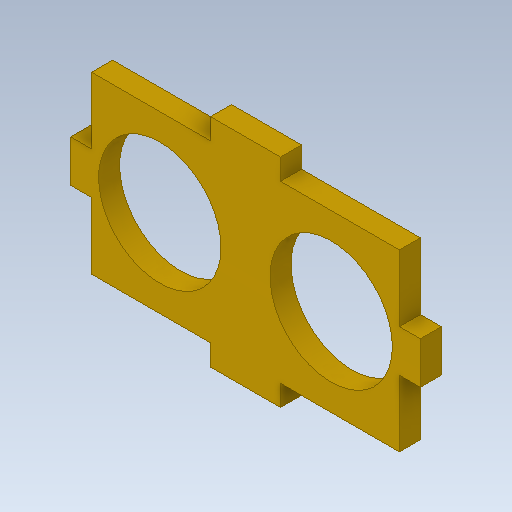
# Autodesk Inventor part: Part5
Saved by Autodesk Inventor 2020 (Build 240168000, 168)
## iProperties
Created: 2020-03-11
Part Number: Part5
Material: Generic
Document SubType Name: Modeling
Designer: tor16003
Density: 1 g/cm^3
Appearance: Gold
Author: tor16003
Autodesk Inventor part; units mm, degrees
ref_plane "YZ Plane" through (0, 0, 0) normal (1, 0, 0) x (0, 1, 0)
ref_plane "XZ Plane" through (0, 0, 0) normal (0, 1, 0) x (-1, 0, 0)
ref_plane "XY Plane" through (0, 0, 0) normal (0, 0, 1) x (1, 0, 0)
sketch "Sketch1" plane through (0, 0, 0) normal (0, 0, 1) x (1, 0, 0)
  line L0 (0, 9.5) -> (-3, 9.5)
  line L1 (-3, 9.5) -> (-3, 15.5)
  line L2 (-3, 15.5) -> (0, 15.5)
  line L3 (0, 15.5) -> (0, 25)
  line L4 (44, 25) -> (44, 15.5)
  line L5 (44, 15.5) -> (47, 15.5)
  line L6 (47, 15.5) -> (47, 9.5)
  line L7 (47, 9.5) -> (44, 9.5)
  line L8 (44, 9.5) -> (44, 0)
  line L9 (0, 0) -> (0, 9.5)
  line L10 (0, 25) -> (17, 25)
  line L11 (17, 25) -> (17, 28)
  line L12 (17, 28) -> (27, 28)
  line L13 (27, 28) -> (27, 25)
  line L14 (27, 25) -> (44, 25)
  line L15 (0, 0) -> (17, 0)
  line L16 (17, 0) -> (17, -3)
  line L17 (17, -3) -> (27, -3)
  line L18 (27, -3) -> (27, 0)
  line L19 (27, 0) -> (44, 0)
  circle A0 centre (9.75, 12.5) radius 8.75
  circle A1 centre (34.25, 12.5) radius 8.75
  line L20 (18.5, 12.5) -> (25.5, 12.5)
  line L21 (-3, 12.5) -> (9.75, 12.5)
  line L22 (34.25, 12.5) -> (47, 12.5)
  dimension "d17" = 17.5
  dimension "d18" = 17.5
  dimension "d2" = 6
  dimension "d3" = 3
  dimension "d7" = 3
  dimension "d8" = 6
  dimension "d12" = 50
  dimension "d13" = 3
  dimension "d14" = 10
  dimension "d15" = 3
  dimension "d19" = 7
  dimension "d22" = 25
  constraints: 46 end point, 13 perpendicular, 7 point on line, 5 equal length, 4 horizontal alignment, 3 collinear, 3 horizontal, 2 midpoint, 1 coincident, 1 vertical, 4 other
  measures "d2" distance of L0.end L1.end
  measures "d3" distance of L1.end L2.end
  measures "d7" distance of L4.end L5.end
  measures "d8" distance of L5.end L6.end
  measures "d12" distance between parallel lines of L6 L1
  measures "d13" distance of L10.end L11.end
  measures "d14" distance between parallel lines of L13 L11
  measures "d15" distance of L15.end L16.end
  measures "d19" distance of L20.start L20.end
  measures "d22" distance between parallel lines of L15 L10
extrude "Extrusion1" add sketch "Sketch1" along normal blind 3 contours L0 L1 L21 A0 L20 A1 L22 L6 L7 L8 L19 L18 L17 L16 L15 L9 | L1 L2 L3 L10 L11 L12 L13 L14 L4 L5 L6 L22 A1 L20 A0 L21
body "Solid1"
